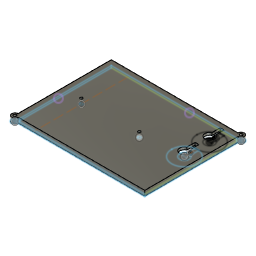
parking_sensor_housing (Autodesk Fusion 360 design; units mm, degrees)
Autodesk Fusion 360 part; units mm, degrees
note: some values were not read from the file. Set by a fixed rule: which sketch regions a step uses.
sketch "Schizzo1" plane through (0, 0, 0) normal (0, 0, 1) x (1, 0, 0)
  line L0 (31, -21) -> (-31, -21)
  line L1 (-31, -21) -> (-31, 21)
  line L2 (-31, 21) -> (31, 21)
  line L3 (31, 21) -> (31, -21)
  line L4 (31, -21) -> (-31, 21) construction
  line L5 (-31, -21) -> (31, 21) construction
  line L6 (32.5, -22.5) -> (-32.5, -22.5)
  line L7 (-32.5, -22.5) -> (-32.5, 22.5)
  line L8 (-32.5, 22.5) -> (32.5, 22.5)
  line L9 (32.5, 22.5) -> (32.5, -22.5)
  line L10 (32.5, -22.5) -> (-32.5, 22.5) construction
  line L11 (-32.5, -22.5) -> (32.5, 22.5) construction
  line L12 (27.5, 17.5) -> (-27.5, 17.5) construction
  line L13 (-27.5, 17.5) -> (-27.5, -17.5) construction
  line L14 (-27.5, -17.5) -> (27.5, -17.5) construction
  line L15 (27.5, -17.5) -> (27.5, 17.5) construction
  line L16 (27.5, 17.5) -> (-27.5, -17.5) construction
  line L17 (-27.5, 17.5) -> (27.5, -17.5) construction
  circle A0 centre (-27.5, 17.5) radius 1
  circle A1 centre (27.5, 17.5) radius 1
  circle A2 centre (-27.5, -17.5) radius 1
  circle A3 centre (27.5, -17.5) radius 1
  circle A4 centre (-27.5, 17.5) radius 2.5
  circle A5 centre (27.5, 17.5) radius 2.5
  circle A6 centre (-27.5, -17.5) radius 2.5
  circle A7 centre (27.5, -17.5) radius 2.5
  line L18 (-31, -15) -> (-32.5, -15)
  line L19 (25, 22.5) -> (25, 21)
  line L20 (-25, 21) -> (-25, 22.5)
  line L21 (-31, 15) -> (-32.5, 15)
  line L22 (-32.5, -10.75) -> (-32.5, -15.75)
  line L23 (0, 0) -> (0, -35)
  line L24 (-32.5, -23) -> (-32.5, -15.75)
  circle A8 centre (60, -45.5) radius 2.5
  circle A9 centre (60, -45.5) radius 1
  circle A10 centre (31, -29.5) radius 2.5
  circle A11 centre (31, -29.5) radius 1
  line L25 (69, -52.5) -> (-31, -52.5)
  line L26 (-31, -52.5) -> (-31, -22.5)
  line L27 (-31, -22.5) -> (69, -22.5)
  line L28 (69, -22.5) -> (69, -52.5)
  line L29 (69, -52.5) -> (-31, -22.5) construction
  line L30 (-31, -52.5) -> (69, -22.5) construction
  line L31 (32.5, 21) -> (69, 21)
  line L32 (69, 21) -> (69, -22.5)
  line L33 (69, -22.5) -> (32.5, -22.5)
  line L34 (32.5, -22.5) -> (32.5, 21)
  line L35 (32.5, 22.5) -> (70.5, 22.5)
  line L36 (70.5, 22.5) -> (70.5, -22.5)
  line L37 (70.5, -22.5) -> (70.5, -54)
  line L38 (70.5, -54) -> (-32.5, -54)
  line L39 (-32.5, -54) -> (-32.5, -22.5)
  line L40 (-32.5, 22.5) -> (-39.6797, 22.5) construction
  line L41 (-39.6797, 22.5) -> (-39.6797, -54) construction
  line L42 (-39.6797, -54) -> (-32.5, -54) construction
  line L43 (-32.5, -54) -> (-32.5, 22.5) construction
  line L44 (-44, -15.75) -> (-39.6797, -15.75) construction
  line L45 (-32.5, -10.75) -> (-40.5, -10.75)
  line L46 (-40.5, -10.75) -> (-40.5, -20.75)
  line L47 (-40.5, -20.75) -> (-32.5, -20.75)
  line L48 (-32.5, -20.75) -> (-32.5, -10.75)
  line L49 (-32.5, -10.75) -> (-40.5, -20.75) construction
  line L50 (-40.5, -10.75) -> (-32.5, -20.75) construction
  line L51 (-40.5, -10.75) -> (-37.5, -10.75)
  line L52 (-37.5, -10.75) -> (-37.5, -20.75)
  line L53 (-37.5, -20.75) -> (-40.5, -20.75)
  line L54 (-40.5, -20.75) -> (-40.5, -10.75)
  line L55 (70.5, -22.25) -> (70.5, -17.25)
  line L56 (70.5, -22.25) -> (78.5, -22.25)
  line L57 (75.5, -22.25) -> (75.5, -12.25)
  line L58 (70.5, -12.25) -> (70.5, -22.25)
  line L59 (78.5, -12.25) -> (70.5, -12.25)
  line L60 (70.5, -22.25) -> (78.5, -12.25) construction
  line L61 (78.5, -22.25) -> (78.5, -12.25)
  line L62 (75.5, -12.25) -> (78.5, -12.25)
  line L63 (78.5, -22.25) -> (70.5, -12.25) construction
  line L64 (78.5, -12.25) -> (78.5, -22.25)
  line L65 (78.5, -22.25) -> (75.5, -22.25)
  line L66 (-25, -21) -> (25, -21)
  line L67 (25, -21) -> (25, -22.5)
  line L68 (25, -22.5) -> (-25, -22.5)
  line L69 (-25, -22.5) -> (-25, -21)
  line L70 (31, 15) -> (32.5, 15)
  line L71 (32.5, 15) -> (32.5, -15)
  line L72 (32.5, -15) -> (31, -15)
  line L73 (31, -15) -> (31, 15)
  circle A12 centre (70.5, 22.5) radius 1
  circle A13 centre (70.5, 22.5) radius 2.5
  circle A14 centre (-32.5, -54) radius 1
  circle A15 centre (-32.5, -54) radius 2.5
  point P0 (19, -37.5)
  point P1 (-36.5, -15.75)
  point P2 (74.5, -17.25)
  dimension "d1" = 62
  dimension "d2" = 42
  dimension "d4" = 1.5
  dimension "d5" = 1.5
  dimension "d6" = 35
  dimension "d7" = 55
  dimension "d8" = 2
  dimension "d11" = 55
  dimension "d12" = 35
  dimension "d13" = 5
  dimension "d16" = 55
  dimension "d17" = -35
  dimension "d44" = 100
  dimension "d45" = 30
  dimension "d46" = 29
  dimension "d47" = 16
  dimension "d48" = 9
  dimension "d49" = 7
  dimension "d52" = 8
  dimension "d53" = 10
  dimension "d54" = 3
  dimension "d55" = 8
  dimension "d56" = 10
  dimension "d57" = 3
  dimension "d69" = 2
  dimension "d70" = 5
  dimension "d71" = 2
  dimension "d72" = 5
  constraint horizontal L0
  constraint perpendicular L0 L1
  constraint parallel L0 L2
  constraint parallel L1 L3
  constraint coincident L4 L23.start
  constraint coincident L5 L23.start
  constraint coincident L23.start origin
  constraint horizontal L6
  constraint perpendicular L6 L7
  constraint parallel L6 L8
  constraint parallel L7 L9
  constraint coincident L10 L23.start
  constraint coincident L11 L23.start
  constraint horizontal L12
  constraint perpendicular L12 L13
  constraint parallel L12 L14
  constraint parallel L13 L15
  constraint coincident L16 L23.start
  constraint coincident L17 L23.start
  constraint coincident L12.end L13.start
  constraint concentric A0 A4
  constraint coincident L1 L18.start
  constraint coincident L7 L18.end
  constraint perpendicular L7 L18
  constraint tangent A6 L18
  constraint coincident L8 L19.start
  constraint coincident L2 L19.end
  constraint perpendicular L8 L19
  constraint tangent A5 L19
  constraint coincident L2 L20.start
  constraint coincident L8 L20.end
  constraint perpendicular L8 L20
  constraint tangent A4 L20
  constraint coincident L1 L21.start
  constraint coincident L7 L21.end
  constraint perpendicular L7 L21
  constraint tangent A4 L21
  constraint vertical L22
  constraint vertical L23
  constraint horizontal L25
  constraint perpendicular L25 L26
  constraint parallel L25 L27
  constraint parallel L26 L28
  constraint coincident L29 P0
  constraint coincident L30 P0
  constraint collinear L6 L27
  constraint collinear L1 L26
  constraint horizontal L31
  constraint vertical L32
  constraint horizontal L33
  constraint vertical L34
  constraint coincident L9 L31.start
  constraint coincident A8.centre A9.centre
  constraint coincident A10.centre A11.centre
  constraint horizontal L40
  constraint vertical L41
  constraint horizontal L42
  constraint vertical L43
  constraint coincident L41 L44.end
  constraint perpendicular L41 L44
  constraint midpoint L41 L44.end
  constraint collinear L38 L42
  constraint horizontal L45
  constraint perpendicular L45 L46
  constraint parallel L45 L47
  constraint parallel L46 L48
  constraint coincident L49 P1
  constraint coincident L50 P1
  constraint collinear L24 L48
  constraint collinear L7 L48
  constraint horizontal L51
  constraint vertical L52
  constraint horizontal L53
  constraint vertical L54
  constraint perpendicular L56 L61
  constraint parallel L56 L59
  constraint parallel L58 L61
  constraint coincident P2 L60
  constraint coincident P2 L63
  constraint horizontal L66
  constraint vertical L67
  constraint horizontal L68
  constraint vertical L69
  constraint coincident L27 L67.end
  constraint coincident L6 L67.end
  constraint coincident L0 L66.start
  constraint tangent A7 L67
  constraint tangent A6 L69
  constraint horizontal L70
  constraint vertical L71
  constraint horizontal L72
  constraint vertical L73
  constraint coincident L34 L71.end
  constraint coincident L3 L70.start
  constraint tangent A5 L70
  constraint tangent A7 L72
  constraint coincident L35.end L36.start
  constraint concentric A12 A13
  constraint coincident L38.end L39.start
  measures "d1" distance of L1.end L2.end
  measures "d2" distance of L0.end L1.end
  measures "d4" distance of L3 L9
  measures "d5" distance of L2 L8
  measures "d6" distance of L12.start L14.end
  measures "d7" distance of L12.start L12.end
  measures "d8" diameter of A0
  measures "d13" diameter of A4
  measures "d44" distance of L26.end L27.end
  measures "d45" distance of L25 L27
  measures "d46" horizontal distance of A8.centre A10.centre
  measures "d47" vertical distance of A8.centre A10.centre
  measures "d48" distance of A8.centre L28
  measures "d49" distance of A8.centre L25
  measures "d52" distance of L46.end L47.end
  measures "d53" distance of L45.end L46.end
  measures "d54" distance of L45.end L51.end
  measures "d55" distance of L59.start L58.start
  measures "d56" distance of L56.end L59.start
  measures "d57" distance of L56.end L57.start
  measures "d69" diameter of A12
  measures "d70" diameter of A13
  measures "d71" diameter of A14
  measures "d72" diameter of A15
extrude "Estrusione1" add sketch "Schizzo1" along normal blind 2 contours L0 L3 L6 L9 L27 L34 L67 L72 | L0 L1 L2 L3 L66 L73 | L0 L6 L23 L27 L66 L67 L68 | L3 L9 L34 L70 L71 L72 L73 | L0 L6 L23 L27 L66 L68 L69 | L6 L25 L26 L27 L28 L33 L68 A15 | L2 L3 L8 L9 L19 L34 L70 | L9 L27 L31 L32 L33 L34 L71 A13 | L0 L1 L6 L7 L18 L22 L24 L27 L48 L69 | L25 L28 L32 L36 L37 L38 L55 L58 A13 A15 | L2 L8 L19 L20 | L9 L31 L35 A13 | L1 L7 L18 L21 L22 L48 | L6 L24 L26 L39 A15 | L31 L32 A13 | L31 L32 L35 L36 A12 A13 | L1 L2 L7 L8 L20 L21 | L25 L26 A15 | L25 L26 L38 L39 A14 A15 | L35 L36 A12 | L38 L39 A14 | A4 | A5 | A6 | A7 | A8 | A10 picked at (70.3587, 21.8502) picked at (-32.1015, -53.4677) makes body 1
extrude "Estrusione2" add sketch "Schizzo1" along normal blind 5 from surface at 2 contours A4 | A5 | A6 | A7 bodies 1
extrude "Estrusione3" add sketch "Schizzo1" along normal blind 7 from surface at 2 separate body contours L0 L3 L6 L9 L27 L34 L67 L72 | L0 L6 L23 L27 L66 L67 L68 | L3 L9 L34 L70 L71 L72 L73 | L0 L6 L23 L27 L66 L68 L69 | L2 L3 L8 L9 L19 L34 L70 | L0 L1 L6 L7 L18 L22 L24 L27 L48 L69 | L25 L28 L32 L36 L37 L38 L55 L58 A13 A15 | L2 L8 L19 L20 | L9 L31 L35 A13 | L1 L7 L18 L21 L22 L48 | L6 L24 L26 L39 A15 | L31 L32 L35 L36 A12 A13 | L1 L2 L7 L8 L20 L21 | L25 L26 L38 L39 A14 A15 | L35 L36 A12 | L38 L39 A14 picked at (70.3587, 21.8502) picked at (-32.1015, -53.4677) makes body 2
extrude "Estrusione7" add sketch "Schizzo1" along normal blind 2 from surface at 2 contours A8 | A10 bodies 1
extrude "Estrusione4" add sketch "Schizzo1" along normal blind 10 from surface at 9 separate body contours L0 L3 L6 L9 L27 L34 L67 L72 | L2 L3 L8 L9 L19 L34 L70 | L0 L1 L6 L7 L18 L22 L24 L27 L48 L69 | L25 L28 L32 L36 L37 L38 L55 L58 A13 A15 | L9 L31 L35 A13 | L6 L24 L26 L39 A15 | L31 L32 L35 L36 A12 A13 | L1 L2 L7 L8 L20 L21 | L25 L26 L38 L39 A14 A15 | L35 L36 A12 | L38 L39 A14 picked at (70.3587, 21.8502) picked at (-32.1015, -53.4677) makes body 3 at (-30, 22.5, 12.3333) makes body 4 at (36.1667, -54, 12.3333) makes body 5 at (32.5, -17.5, 12.3333)
extrude "Estrusione8" add sketch "Schizzo1" along normal blind 5 contours L7 L22 L24 L45 L47 L48 L52 | L36 L55 L56 L57 L58 L59 | L45 L46 L47 L51 L52 L53 L54 | L56 L57 L59 L61 L62 L64 L65 bodies 1 3 4 5 2
extrude "Estrusione9" add sketch "Schizzo1" along normal blind 3 from surface at 5 contours L45 L46 L47 L51 L52 L53 L54 | L56 L57 L59 L61 L62 L64 L65 bodies 1
chamfer "Smusso2" distance 3 angle 45 8 edges at (73, -12.25, 5) (77, -12.25, 8) (77, -22.25, 8) (73, -22.25, 5) (-35, -20.75, 5) (-39, -20.75, 8) (-35, -10.75, 5) (-39, -10.75, 8) on bodies 1
extrude "Estrusione10" add sketch "Schizzo1" against normal blind 3 from surface at 19 contours L35 L36 A12 A13 | L38 L39 A14 A15 bodies 4
extrude "Estrusione11" cut sketch "Schizzo1" against normal blind 5 from surface at 19 contours L35 L36 A12 | L35 L36 A12 | L38 L39 A14 | L38 L39 A14 bodies 4
sketch "Schizzo1 (2)" plane through (0, 0, 2) normal (0, 0, 1) x (-1, 0, 0) in component "top"
  line L0 (31, -21) -> (31, 21)
  line L1 (-31, -21) -> (31, -21)
  circle A0 centre (-70.5, -22.5) radius 2.5
  circle A1 centre (-70.5, -22.5) radius 1.15
  circle A2 centre (32.5, 54) radius 2.5
  circle A3 centre (32.5, 54) radius 1.15
  line L2 (32.5, 54) -> (-70.5, 54)
  line L3 (-70.5, 54) -> (-70.5, -22.5)
  line L4 (-70.5, -22.5) -> (32.5, -22.5)
  line L5 (32.5, -22.5) -> (32.5, 54)
  line L6 (31, 52.5) -> (-69, 52.5)
  line L7 (-69, 52.5) -> (-69, -21)
  line L8 (-69, -21) -> (31, -21)
  line L9 (31, -21) -> (31, 52.5)
  circle A4 centre (-59, -9) radius 3.75
  line L10 (-60.5, -9) -> (-57.5, -9)
  line L11 (-57.5, -9) -> (-57.5, -19)
  line L12 (-57.5, -19) -> (-60.5, -19)
  line L13 (-60.5, -19) -> (-60.5, -9)
  line L14 (-60.5, -9) -> (-57.5, -19) construction
  line L15 (-57.5, -9) -> (-60.5, -19) construction
  circle A5 centre (-59, -9) radius 10
  line L16 (-60.5, 11) -> (-57.5, 1) construction
  line L17 (-60.5, 11) -> (-57.5, 11)
  circle A6 centre (-59, 11) radius 10
  line L18 (-57.5, 11) -> (-57.5, 1)
  line L19 (-57.5, 1) -> (-60.5, 1)
  line L20 (-57.5, 11) -> (-60.5, 1) construction
  circle A7 centre (-59, 11) radius 3.75
  line L21 (-60.5, 1) -> (-60.5, 11)
  circle A8 centre (18, 15.75) radius 1
  circle A9 centre (-28, 15.75) radius 1
  line L22 (18, -21) -> (18, 52.5) construction
  point P0 (-59, -14)
  point P1 (-59, 6)
  dimension "d79" = 5
  dimension "d80" = 2.3
  dimension "d81" = 5
  dimension "d82" = 2.3
  dimension "d83" = 7.5
  dimension "d84" = 3
  dimension "d85" = 10
  dimension "d86" = 12
  dimension "d87" = 20
  dimension "d88" = 7.5
  dimension "d89" = 3
  dimension "d90" = 10
  dimension "d91" = 20
  dimension "d92" = 20
  dimension "d93" = 10
  dimension "d99" = 2
  dimension "d100" = 2
  dimension "d101" = 46
  constraint concentric A0 A1
  constraint concentric A2 A3
  constraint horizontal L2
  constraint vertical L3
  constraint horizontal L4
  constraint vertical L5
  constraint coincident A0.centre A1.centre
  constraint coincident A2.centre A3.centre
  constraint horizontal L6
  constraint vertical L7
  constraint horizontal L8
  constraint vertical L9
  constraint horizontal L10
  constraint perpendicular L10 L11
  constraint parallel L10 L12
  constraint parallel L11 L13
  constraint coincident L14 P0
  constraint coincident L15 P0
  constraint midpoint A4.centre L10
  constraint concentric A4 A5
  constraint horizontal L17
  constraint perpendicular L17 L18
  constraint parallel L17 L19
  constraint parallel L18 L21
  constraint coincident P1 L16
  constraint coincident P1 L20
  constraint midpoint A6.centre L17
  constraint concentric A6 A7
  constraint coincident L8 L22.start
  constraint coincident L6 L22.end
  constraint perpendicular L6 L22
  constraint midpoint A8.centre L22
  measures "d79" diameter of A0
  measures "d80" diameter of A1
  measures "d81" diameter of A2
  measures "d82" diameter of A3
  measures "d83" diameter of A4
  measures "d84" distance of L11.end L12.end
  measures "d85" distance of L10.end L11.end
  measures "d86" distance of L8 A4.centre
  measures "d87" diameter of A5
  measures "d88" diameter of A7
  measures "d89" distance of L19.end L16.end
  measures "d90" distance of L17.end L16.end
  measures "d91" diameter of A6
  measures "d92" distance of A4.centre A6.centre
  measures "d93" distance of L7 A4.centre
  measures "d99" diameter of A8
  measures "d100" diameter of A9
  measures "d101" distance of A8.centre A9.centre
extrude "Estrusione1'" add sketch "Schizzo1 (2)" along normal blind 2 separate body contours L0 L1 A0 A2 L4 L5 L8 L9 | A2 A3 L2 L5 L6 L9 | A2 L6 L9 | A0 L7 L8 | A0 A1 L3 L4 L7 L8 | A0 A2 L2 L3 L6 L7 | A2 A3 L2 L5 | A0 A1 L3 L4 makes body 6 in component "top"
extrude "Estrusione2'" add sketch "Schizzo1 (2)" along normal blind 2 from surface at 2 contours L0 L1 A0 A2 L6 L7 L8 L9 L11 L12 L13 A5 A6 L18 L19 | L0 L1 A0 A2 L4 L5 L8 L9 | A2 A3 L2 L5 L6 L9 | A2 L6 L9 | A0 L7 L8 | A0 A1 L3 L4 L7 L8 | A0 A2 L2 L3 L6 L7 | A2 A3 L2 L5 | A0 A1 L3 L4 | L7 A5 A6 L19 L21 | A4 L11 L13 A5 | A6 L18 A7 L21 | A6 L19 L21 | A6 L18 L19 | L12 L13 A5 | L11 L12 A5 | A8 | A9 picked at (-61.7609, -1.5985) picked at (-66.879, 11.5308) bodies 6 in component "top"
extrude "Estrusione3'" cut sketch "Schizzo1 (2)" along normal blind 4 contours A8 | A9 bodies 6 in component "top"
component "top" placed x (1, 0, 0) y (0, 1, 0) z (0, 0, 1) at (0, 0, 0)
equation "wall_thickness = 1.5 mm"
equation "d4 = wall_thickness"
equation "d5 = wall_thickness"
equation "d50 = -wall_thickness"
